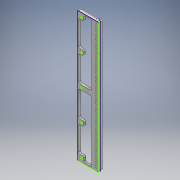
# Autodesk Inventor part: LDR_Holder_1
Saved by Autodesk Inventor 2017 (Build 210142000, 142)
## iProperties
Created: 2017-05-03
Part Number: LDR_Holder_1
Material: Generic
Document SubType Name: Modeling
Designer: willt
Density: 1 g/cm^3
Appearance: Default
Author: willt
Autodesk Inventor part; units mm, degrees
ref_plane "YZ Plane" through (0, 0, 0) normal (1, 0, 0) x (0, 1, 0)
ref_plane "XZ Plane" through (0, 0, 0) normal (0, 1, 0) x (-1, 0, 0)
ref_plane "XY Plane" through (0, 0, 0) normal (0, 0, 1) x (1, 0, 0)
sketch "Sketch1" plane through (0, 0, 0) normal (0, 1, 0) x (-1, 0, 0)
  line L0 (0, 0) -> (-50.5, 0)
  line L1 (-50.5, 0) -> (-50.5, -312.6)
  line L2 (-50.5, -312.6) -> (0, -312.6)
  line L3 (0, -312.6) -> (0, 0)
  circle A0 centre (-10, -10) radius 2.625
  circle A1 centre (-10, -156.3) radius 2.625
  circle A2 centre (-10, -302.6) radius 2.625
  circle A3 centre (-10, -229.45) radius 2.625
  circle A4 centre (-10, -83.15) radius 2.625
  constraints: 8 end point, 5 centre point, 2 parallel, 1 horizontal, 1 perpendicular
extrude "Extrusion1" add sketch "Sketch1" along normal blind 5 contours L3 L2 L1 L0 | A3 | A4
sketch "Sketch2" plane through (0, 5, 0) normal (0, 1, 0) x (1, 0, 0)
  line L0 (0, 0) -> (50.5, 0) construction
  line L1 (45, 0) -> (45, 312.6) construction
  line L2 (50.5, 312.6) -> (0, 312.6) construction
  line L3 (0, 312.6) -> (0, 0) construction
  circle A0 centre (43.3, 5.1) radius 0.5
  circle A1 centre (46.7, 5.1) radius 0.5
  line L4 (50.5, 0) -> (48, 0)
  line L5 (48, 0) -> (48, 312.6)
  line L6 (48, 312.6) -> (50.5, 312.6)
  line L7 (50.5, 312.6) -> (50.5, 0)
  line L8 (42, 0) -> (39.5, 0)
  line L9 (39.5, 0) -> (39.5, 312.6)
  line L10 (39.5, 312.6) -> (42, 312.6)
  line L11 (42, 312.6) -> (42, 0)
  constraints: 18 end point, 4 parallel, 3 point on line, 2 centre point, 2 horizontal, 2 perpendicular, 1 vertical
extrude "Extrusion2" cut sketch "Sketch2" against normal blind 5 contours A0 | A1
pattern_linear "Rectangular Pattern1" count 71 spacing 4.3 along (0, 0, -1) of "Extrusion2"
extrude "Extrusion3" add sketch "Sketch2" along normal blind 5.25 contours L4 L5 L6 L7 | L8 L9 L10 L11
sketch "Sketch3" plane through (0, 0, 0) normal (0, 0, 1) x (1, 0, 0)
  line L0 (39.5, 5) -> (34, 5)
  line L1 (0, 5) -> (39.5, 5) projected
  line L2 (34, 5) -> (39.5, 10.25)
  line L3 (39.5, 10.25) -> (39.5, 5)
  point P0 (0, 0)
  dimension "d37" = 5.5
  constraints: 6 end point, 1 perpendicular, 1 point on line
  measures "d37" distance of L0.start L0.end
extrude "Extrusion4" add sketch "Sketch3" against normal blind 312.6
fillet "Fillet1" radius 2 1 edges at (39.5, 10.25, -156.3)
sketch "Sketch4" plane through (0, 0, 0) normal (0, -1, 0) x (1, 0, 0)
  line L0 (0, -312.6) -> (0, 0) projected
  line L1 (0, -156.3) -> (50.5, -156.3)
  line L2 (50.5, 0) -> (50.5, -312.6) projected
  circle A0 centre (10, -302.6) radius 2.625 construction
  line L3 (10, -299.975) -> (10, -296.975) construction
  line L4 (12.625, -302.6) -> (15.625, -302.6) construction
  line L5 (50.5, -312.6) -> (0, -312.6) construction
  line L6 (15.625, -312.6) -> (15.625, -309.6) construction
  circle A1 centre (10, -156.3) radius 2.625 construction
  line L7 (10, -158.925) -> (10, -161.925) construction
  line L8 (0, -312.6) -> (0, 0) construction
  line L9 (0, -296.975) -> (3, -296.975) construction
  circle A2 centre (10, -10) radius 2.625 construction
  line L10 (12.625, -10) -> (15.625, -10) construction
  line L11 (15.625, 0) -> (15.625, -3) construction
  line L12 (10, -153.675) -> (10, -150.675) construction
  line L13 (50.5, -309.6) -> (34, -309.6) construction
  line L14 (15.625, -306.6) -> (15.625, -302.6)
  line L15 (12.625, -296.975) -> (10, -296.975)
  line L16 (15.625, -302.6) -> (15.625, -299.975)
  line L17 (10, -296.975) -> (6, -296.975)
  line L18 (18.625, -309.6) -> (31, -309.6)
  line L19 (10, -161.925) -> (6, -161.925)
  line L20 (10, -161.925) -> (31, -161.925)
  line L21 (34, -164.925) -> (34, -306.6)
  line L22 (15.625, -10) -> (15.625, -6)
  line L23 (0, 0) -> (50.5, 0) projected
  line L24 (18.625, -3) -> (31, -3)
  line L25 (34, -6) -> (34, -147.675)
  line L26 (31, -150.675) -> (10, -150.675)
  line L27 (10, -150.675) -> (6, -150.675)
  line L28 (10, -12.625) -> (10, -15.625) construction
  line L29 (15.625, -10) -> (15.625, -12.625)
  line L30 (12.625, -15.625) -> (10, -15.625)
  line L31 (10, -15.625) -> (6, -15.625)
  circle A3 centre (10, -83.15) radius 2.625
  circle A4 centre (10, -229.45) radius 2.625
  line L32 (10, -232.075) -> (10, -235.075) construction
  line L33 (10, -226.825) -> (10, -223.825) construction
  line L34 (10, -85.775) -> (10, -88.775) construction
  line L35 (10, -80.525) -> (10, -77.525) construction
  line L36 (10, -235.075) -> (6, -235.075)
  line L37 (3, -238.075) -> (3, -293.975)
  line L38 (10, -235.075) -> (12.625, -235.075)
  line L39 (15.625, -232.075) -> (15.625, -226.825)
  line L40 (12.625, -223.825) -> (6, -223.825)
  line L41 (3, -220.825) -> (3, -164.925)
  line L42 (10, -88.775) -> (6, -88.775)
  line L43 (3, -91.775) -> (3, -147.675)
  line L44 (10, -77.525) -> (6, -77.525)
  line L45 (3, -74.525) -> (3, -18.625)
  line L46 (10, -88.775) -> (11.125, -88.775)
  line L47 (14.125, -85.775) -> (14.125, -80.525)
  line L48 (11.125, -77.525) -> (10, -77.525)
  arc A5 (3, -293.975) -> (6, -296.975) centre (6, -293.975) ccw
  arc A6 (15.625, -299.975) -> (12.625, -296.975) centre (12.625, -299.975) ccw
  arc A7 (15.625, -306.6) -> (18.625, -309.6) centre (18.625, -306.6) ccw
  arc A8 (31, -309.6) -> (34, -306.6) centre (31, -306.6) ccw
  arc A9 (6, -235.075) -> (3, -238.075) centre (6, -238.075) ccw
  arc A10 (12.625, -235.075) -> (15.625, -232.075) centre (12.625, -232.075) ccw
  arc A11 (15.625, -226.825) -> (12.625, -223.825) centre (12.625, -226.825) ccw
  arc A12 (3, -220.825) -> (6, -223.825) centre (6, -220.825) ccw
  arc A13 (6, -161.925) -> (3, -164.925) centre (6, -164.925) ccw
  arc A14 (34, -164.925) -> (31, -161.925) centre (31, -164.925) ccw
  arc A15 (31, -150.675) -> (34, -147.675) centre (31, -147.675) ccw
  arc A16 (3, -147.675) -> (6, -150.675) centre (6, -147.675) ccw
  arc A17 (6, -88.775) -> (3, -91.775) centre (6, -91.775) ccw
  arc A18 (11.125, -88.775) -> (14.125, -85.775) centre (11.125, -85.775) ccw
  arc A19 (14.125, -80.525) -> (11.125, -77.525) centre (11.125, -80.525) ccw
  arc A20 (3, -74.525) -> (6, -77.525) centre (6, -74.525) ccw
  arc A21 (6, -15.625) -> (3, -18.625) centre (6, -18.625) ccw
  arc A22 (12.625, -15.625) -> (15.625, -12.625) centre (12.625, -12.625) ccw
  arc A23 (18.625, -3) -> (15.625, -6) centre (18.625, -6) ccw
  arc A24 (34, -6) -> (31, -3) centre (31, -6) ccw
  point P0 (15.625, -296.975)
  point P1 (3, -150.675)
  point P2 (3, -15.625)
  point P3 (15.625, -235.075)
  point P4 (3, -223.825)
  point P5 (3, -88.775)
  point P6 (3, -77.525)
  point P7 (14.125, -88.775)
  point P8 (14.125, -77.525)
  dimension "d65" = 16.5
  dimension "d69" = 73.15
  dimension "d71" = 73.15
  dimension "d72" = 3
  dimension "d73" = 3
  dimension "d74" = 3
  dimension "d75" = 3
  dimension "d76" = 3
  constraints: 88 end point, 50 point on circle, 40 tangent, 38 point on line, 22 centre point, 19 equal radius, 17 perpendicular, 13 vertical, 7 horizontal, 2 midpoint, 1 collinear
  measures "d65" distance of L13.start L13.end
  measures "d69" distance of A3.centre A2.centre
  measures "d71" distance of A0.centre A4.centre
  measures "d72" distance of L32.start L32.end
  measures "d73" distance of L33.start L33.end
  measures "d74" distance of L34.start L34.end
  measures "d75" distance of L35.start L35.end
  measures "d76" radius of A5
extrude "Extrusion5" cut sketch "Sketch1" along normal blind 5 contours A4
extrude "Extrusion6" cut sketch "Sketch1" along normal up to next contours A3
extrude "Extrusion7" cut sketch "Sketch4" against normal up to next contours L14 L16 A6 L15 L17 A5 L37 A9 L36 L38 A10 L39 A11 L40 A12 L41 A13 L19 L20 A14 L21 A8 L18 A7 | L22 A23 L24 A24 L25 A15 L26 L27 A16 L43 A17 L42 L46 A18 L47 A19 L48 L44 A20 L45 A21 L31 L30 A22 L29
fillet "Fillet2" radius 3 4 edges at (0, 2.5, -312.6) (50.5, 5.125, -312.6) (50.5, 5.125, 0) (0, 2.5, 0)
body "Solid1"
